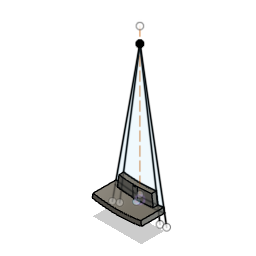
Food_proc_part v2 (Autodesk Fusion 360 design; units mm, degrees)
Autodesk Fusion 360 part; units mm, degrees
note: some values were not read from the file. Chosen so that the rebuilt part matches the saved one: where a step ends.
sketch "Sketch1" plane through (0, 0, 0) normal (0, 0, 1) x (1, 0, 0)
  line L0 (0, 0) -> (13.0703, -95.4158)
  line L1 (0, 0) -> (-13.1844, -96.2486)
  line L2 (0, 10) -> (0, -85) construction
  arc A0 (-10.6537, -77.7737) -> (10.6537, -77.7737) centre (0, 0) ccw
  line L3 (0, 0) -> (17.4117, -94.8691)
  line L4 (0, 0) -> (-17.9563, -97.8361)
  arc A1 (-15.5246, -84.5871) -> (15.5246, -84.5871) centre (0, 0) ccw
  arc A2 (-16.0662, -87.5379) -> (16.0662, -87.5379) centre (0, 0) ccw
  dimension "d1" = 7.8
  dimension "d2" = 7.8
  dimension "d3" = 10.4
  dimension "d4" = 10.4
  dimension "d14" = 78.5
  dimension "d15" = 86
  dimension "d16" = 89
  constraint coincident L0.start L1.start
  constraint vertical L2
  constraint coincident L1 A0.start
  constraint coincident L4 A1.start
  constraint coincident L4 A2.start
  constraint coincident L0 A0.end
  constraint coincident L3 A1.end
  constraint coincident L3 A2.end
  measures "d1" angle of L0 L2
  measures "d2" angle of L1 L2
  measures "d3" angle of L2 L3
  measures "d4" angle of L2 L4
  measures "d14" distance of L0.start A0.start
  measures "d15" distance of L0.start A1.start
  measures "d16" distance of L0.start A2.start
extrude "Extrude1" add sketch "Sketch1" along normal blind 15 contours L0 L3 A1 A2 | L1 L4 A1 A2 | L0 L1 A1 A2
extrude "Extrude2" add sketch "Sketch1" along normal blind 3 contours L0 L1 A0 A1
ref_plane "WorkPlane1" through (0, -88, 0) normal (0, 1, 0) x (0, 0, 1)
sketch "Sketch2" plane through (0, -88, 0) normal (0, 1, 0) x (1, 0, 0)
  circle A0 centre (0, -2.3) radius 1.5
  dimension "d18" = 3
  dimension "d19" = 2.3
  measures "d18" diameter of A0
  measures "d19" distance of A0.centre origin
extrude "Extrude3" add sketch "Sketch2" along normal blind 9.5 and the other way up to far side of body 1
